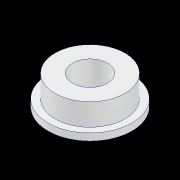
# Autodesk Inventor part: 3MMBearing
Saved by Autodesk Inventor 2021 (Build 250183000, 183)
## iProperties
Created: 2021-03-30
Part Number: 3MMBearing
Material: Aluminum 6061
Document SubType Name: Modeling
Designer: Esketitttttt
Mass: 0.34 g
Surface Area: 1.40241 cm^2
Volume: 0.0604788 cm^3
Density: 2.7 g/cm^3
Appearance: Aluminum - Flat
Author: Esketitttttt
Autodesk Inventor part; units mm, degrees
ref_plane "YZ Plane" through (0, 0, 0) normal (1, 0, 0) x (0, 1, 0)
ref_plane "XZ Plane" through (0, 0, 0) normal (0, 1, 0) x (-1, 0, 0)
ref_plane "XY Plane" through (0, 0, 0) normal (0, 0, 1) x (1, 0, 0)
sketch "Sketch1" plane through (0, 0, 0) normal (0, 1, 0) x (-1, 0, 0)
  circle A0 centre (0, 0) radius 1.5
  circle A1 centre (0, 0) radius 3
  circle A2 centre (0, 0) radius 3.6
  dimension "d0" = 3
  dimension "d1" = 6
  dimension "d2" = 7.2
  constraints: 3 centre point, 3 coincident
  measures "d0" diameter of A0
  measures "d1" diameter of A1
  measures "d2" diameter of A2
extrude "Extrusion1" add sketch "Sketch1" along normal blind 2.5 contours A1
extrude "Extrusion2" add sketch "Sketch1" along normal blind 0.6 contours A2
body "Solid1"
